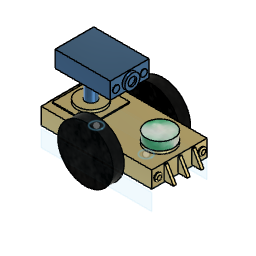
frp_1100309 v2 (Autodesk Fusion 360 design; units mm, degrees)
Autodesk Fusion 360 part; units mm, degrees
sketch "Sketch1" plane through (0, 0, 0) normal (0, 0, 1) x (1, 0, 0)
  line L0 (100, -50) -> (-100, -50)
  line L1 (-100, -50) -> (-100, 50)
  line L2 (-100, 50) -> (100, 50)
  line L3 (100, 50) -> (100, -50)
  line L4 (100, -50) -> (-100, 50) construction
  line L5 (-100, -50) -> (100, 50) construction
  dimension "d1" = 200
  dimension "d2" = 100
  constraint horizontal L0
  constraint perpendicular L0 L1
  constraint parallel L0 L2
  constraint parallel L1 L3
  constraint coincident L4 origin
  constraint coincident L5 origin
  measures "d1" distance of L1.end L2.end
  measures "d2" distance of L0.end L1.end
extrude "Extrude1" add sketch "Sketch1" along normal blind 30 makes body 1
sketch "Sketch2" plane through (0, -50, 0) normal (0, -1, 0) x (1, 0, 0)
  line L0 (-100, 0) -> (100, 0)
  line L1 (100, 0) -> (100, 30)
  line L2 (100, 30) -> (-100, 30)
  line L3 (-100, 30) -> (-100, 0)
sketch "Sketch3" plane through (0, 50, 0) normal (0, 1, 0) x (-1, 0, 0)
  line L0 (-100, 0) -> (100, 0)
  line L1 (100, 0) -> (100, 30)
  line L2 (100, 30) -> (-100, 30)
  line L3 (-100, 30) -> (-100, 0)
  circle A0 centre (0, 15) radius 25
  dimension "d8" = 50
  measures "d8" diameter of A0
sketch "Sketch4" plane through (0, 0, 30) normal (0, 0, 1) x (-1, 0, 0)
  line L0 (-100, -50) -> (100, -50)
  line L1 (100, -50) -> (100, 50)
  line L2 (100, 50) -> (-100, 50)
  line L3 (-100, 50) -> (-100, -50)
  circle A0 centre (-65, 0) radius 25
  dimension "d11" = 50
  measures "d11" diameter of A0
extrude "Extrude4" add sketch "Sketch4" along normal blind 5 contours A0 bodies 1
sketch "Sketch5" plane through (0, 0, 35) normal (0, 0, 1) x (-1, 0, 0)
  circle A0 centre (-65, 0) radius 25
  circle A1 centre (-65, 0) radius 25
  dimension "d14" = 50
  constraint concentric A0 A1
  measures "d14" diameter of A1
extrude "Extrude5" add sketch "Sketch5" along normal blind 15 separate body makes body 2
sketch "Sketch6" plane through (0, 0, 30) normal (0, 0, 1) x (-1, 0, 0)
  circle A0 centre (-65, 0) radius 25
  line L0 (-100, -50) -> (100, -50)
  line L1 (100, -50) -> (100, 50)
  line L2 (100, 50) -> (-100, 50)
  line L3 (-100, 50) -> (-100, -50)
  line L4 (25, 35) -> (95, 35)
  line L5 (95, 35) -> (95, -35)
  line L6 (95, -35) -> (25, -35)
  line L7 (25, -35) -> (25, 35)
  line L8 (25, 35) -> (95, -35) construction
  line L9 (95, 35) -> (25, -35) construction
  point P0 (60, 0)
  dimension "d17" = 70
  dimension "d18" = 70
  constraint horizontal L4
  constraint perpendicular L4 L5
  constraint parallel L4 L6
  constraint parallel L5 L7
  constraint coincident L8 P0
  constraint coincident L9 P0
  measures "d17" distance of L5.end L6.end
  measures "d18" distance of L4.end L5.end
extrude "Extrude6" add sketch "Sketch6" along normal blind 2 contours L4 L5 L6 L7 bodies 1
sketch "Sketch7" plane through (0, 0, 32) normal (0, 0, 1) x (-1, 0, 0)
  line L0 (25, -35) -> (95, -35)
  line L1 (95, -35) -> (95, 35)
  line L2 (95, 35) -> (25, 35)
  line L3 (25, 35) -> (25, -35)
  circle A0 centre (60, 0) radius 25
  dimension "d21" = 50
  measures "d21" diameter of A0
extrude "Extrude7" add sketch "Sketch7" along normal blind 5 contours A0 bodies 1
sketch "Sketch8" plane through (0, 0, 37) normal (0, 0, 1) x (-1, 0, 0)
  circle A0 centre (60, 0) radius 25
  circle A1 centre (60, 0) radius 10
  dimension "d24" = 20
  constraint concentric A0 A1
  measures "d24" diameter of A1
extrude "Extrude8" add sketch "Sketch8" along normal blind 50 separate body contours A1 makes body 3
sketch "Sketch9" plane through (0, 0, 87) normal (0, 0, 1) x (-1, 0, 0)
  circle A0 centre (60, 0) radius 10
  line L0 (-10, -35) -> (90, -35)
  line L1 (90, -35) -> (90, 35)
  line L2 (90, 35) -> (-10, 35)
  line L3 (-10, 35) -> (-10, -35)
  line L4 (-10, -35) -> (90, 35) construction
  line L5 (90, -35) -> (-10, 35) construction
  point P0 (40, 0)
  dimension "d27" = 100
  constraint horizontal L0
  constraint perpendicular L0 L1
  constraint parallel L0 L2
  constraint parallel L1 L3
  constraint coincident L4 P0
  constraint coincident L5 P0
  measures "d27" distance of L1.end L2.end
extrude "Extrude9" add sketch "Sketch9" along normal blind 30 contours A0 | L0 L1 L2 L3 bodies 3
sketch "Sketch10" plane through (10, 0, 0) normal (1, 0, 0) x (0, 1, 0)
  line L0 (-35, 87) -> (35, 87)
  line L1 (35, 87) -> (35, 117)
  line L2 (35, 117) -> (-35, 117)
  line L3 (-35, 117) -> (-35, 87)
  circle A0 centre (0, 101.2139) radius 13.5
  circle A1 centre (-25, 100) radius 6
  circle A2 centre (25, 100) radius 6
  dimension "d30" = 27
  dimension "d31" = 12
  dimension "d32" = 12
  measures "d30" diameter of A0
  measures "d31" diameter of A1
  measures "d32" diameter of A2
extrude "Extrude10" add sketch "Sketch10" along normal blind 2 contours A0 bodies 3
extrude "Extrude11" add sketch "Sketch10" along normal blind 1 contours A1 bodies 3
extrude "Extrude12" add sketch "Sketch10" along normal blind 1 contours A2 bodies 3
sketch "Sketch11" plane through (12, 0, 0) normal (1, 0, 0) x (0, 1, 0)
  circle A0 centre (0, 101.2139) radius 13.5
  circle A1 centre (0, 101.2139) radius 7.5
  dimension "d39" = 15
  constraint concentric A0 A1
  measures "d39" diameter of A1
extrude "Extrude13" add sketch "Sketch11" along normal blind 3 bodies 3
sketch "Sketch12" plane through (100, 0, 0) normal (1, 0, 0) x (0, 1, 0)
  line L0 (-50, 0) -> (50, 0)
  line L1 (50, 0) -> (50, 30)
  line L2 (50, 30) -> (-50, 30)
  line L3 (-50, 30) -> (-50, 0)
  line L4 (-22.5, 2) -> (-27.5, 2)
  line L5 (-27.5, 2) -> (-27.5, 28)
  line L6 (-27.5, 28) -> (-22.5, 28)
  line L7 (-22.5, 28) -> (-22.5, 2)
  line L8 (-22.5, 2) -> (-27.5, 28) construction
  line L9 (-27.5, 2) -> (-22.5, 28) construction
  line L10 (2.5, 2) -> (-2.5, 2)
  line L11 (-2.5, 2) -> (-2.5, 28)
  line L12 (-2.5, 28) -> (2.5, 28)
  line L13 (2.5, 28) -> (2.5, 2)
  line L14 (2.5, 2) -> (-2.5, 28) construction
  line L15 (-2.5, 2) -> (2.5, 28) construction
  line L16 (27.5, 2) -> (22.5, 2)
  line L17 (22.5, 2) -> (22.5, 28)
  line L18 (22.5, 28) -> (27.5, 28)
  line L19 (27.5, 28) -> (27.5, 2)
  line L20 (27.5, 2) -> (22.5, 28) construction
  line L21 (22.5, 2) -> (27.5, 28) construction
  point P0 (-25, 15)
  point P1 (0, 15)
  point P2 (25, 15)
  dimension "d42" = 5
  dimension "d43" = 26
  dimension "d44" = 5
  dimension "d45" = 26
  dimension "d46" = 5
  dimension "d47" = 26
  constraint horizontal L4
  constraint perpendicular L4 L5
  constraint parallel L4 L6
  constraint parallel L5 L7
  constraint coincident L8 P0
  constraint coincident L9 P0
  constraint horizontal L10
  constraint perpendicular L10 L11
  constraint parallel L10 L12
  constraint parallel L11 L13
  constraint coincident L14 P1
  constraint coincident L15 P1
  constraint horizontal L16
  constraint perpendicular L16 L17
  constraint parallel L16 L18
  constraint parallel L17 L19
  constraint coincident L20 P2
  constraint coincident L21 P2
  measures "d42" distance of L5.end L6.end
  measures "d43" distance of L4.end L5.end
  measures "d44" distance of L11.end L12.end
  measures "d45" distance of L10.end L11.end
  measures "d46" distance of L17.end L18.end
  measures "d47" distance of L16.end L17.end
extrude "Extrude14" add sketch "Sketch12" along normal blind 2 contours L4 L5 L6 L7 bodies 1
extrude "Extrude15" add sketch "Sketch12" along normal blind 2 contours L10 L11 L12 L13 bodies 1
extrude "Extrude16" add sketch "Sketch12" along normal blind 2 contours L16 L17 L18 L19 bodies 1
draft "Draft1" angle 30 neutral plane through (100, -27.5, 28) pull (0, 0, 1) 1 faces at (102, -24.1667, 19.3333) on bodies 1
draft "Draft2" angle 30 neutral plane through (100, -2.5, 28) pull (0, 0, 1) 1 faces at (102, -0.8333, 10.6667) on bodies 1
draft "Draft3" angle 30 neutral plane through (100, 22.5, 28) pull (0, 0, 1) 1 faces at (102, 25.8333, 19.3333) on bodies 1
sketch "Sketch13" plane through (100, 0, 0) normal (1, 0, 0) x (0, 1, 0)
  circle A0 centre (-40, 15) radius 6.5
  circle A1 centre (40, 15) radius 6.5
  dimension "d60" = 13
  dimension "d61" = 13
  measures "d60" diameter of A0
  measures "d61" diameter of A1
extrude "Extrude17" add sketch "Sketch13" along normal blind 4 contours A0 bodies 1
extrude "Extrude18" add sketch "Sketch13" along normal blind 4 contours A1 bodies 1
fillet "Fillet1" radius 2.5 tangency weight 1.76356 1 faces at (104, -41.5883, 13.5263) on bodies 1
fillet "Fillet2" radius 2.5 1 faces at (104, 38.4117, 13.5263) on bodies 1
sketch "Sketch14" plane through (-100, 0, 0) normal (-1, 0, 0) x (0, -1, 0)
  line L0 (-50, 0) -> (50, 0)
  line L1 (50, 0) -> (50, 30)
  line L2 (50, 30) -> (-50, 30)
  line L3 (-50, 30) -> (-50, 0)
  line L4 (35, 26.5) -> (-35, 26.5)
  line L5 (-35, 26.5) -> (-35, 3.5)
  line L6 (-35, 3.5) -> (35, 3.5)
  line L7 (35, 3.5) -> (35, 26.5)
  line L8 (35, 26.5) -> (-35, 3.5) construction
  line L9 (-35, 26.5) -> (35, 3.5) construction
  point P0 (0, 15)
  dimension "d70" = 70
  dimension "d71" = 23
  constraint horizontal L4
  constraint perpendicular L4 L5
  constraint parallel L4 L6
  constraint parallel L5 L7
  constraint coincident L8 P0
  constraint coincident L9 P0
  measures "d70" distance of L5.end L6.end
  measures "d71" distance of L4.end L5.end
extrude "Extrude19" add sketch "Sketch14" along normal blind 2 contours L4 L5 L6 L7 bodies 1
sketch "Sketch15" plane through (-102, 0, 0) normal (-1, 0, 0) x (0, -1, 0)
  line L0 (35, 3.5) -> (35, 26.5)
  line L1 (35, 26.5) -> (-35, 26.5)
  line L2 (-35, 26.5) -> (-35, 3.5)
  line L3 (-35, 3.5) -> (35, 3.5)
  line L4 (-18, 6) -> (-22, 6)
  line L5 (-22, 6) -> (-22, 24)
  line L6 (-22, 24) -> (-18, 24)
  line L7 (-18, 24) -> (-18, 6)
  line L8 (-18, 6) -> (-22, 24) construction
  line L9 (-22, 6) -> (-18, 24) construction
  line L10 (2, 24) -> (-2, 24)
  line L11 (-2, 24) -> (-2, 6)
  line L12 (-2, 6) -> (2, 6)
  line L13 (2, 6) -> (2, 24)
  line L14 (2, 24) -> (-2, 6) construction
  line L15 (-2, 24) -> (2, 6) construction
  line L16 (22, 6) -> (18, 6)
  line L17 (18, 6) -> (18, 24)
  line L18 (18, 24) -> (22, 24)
  line L19 (22, 24) -> (22, 6)
  line L20 (22, 6) -> (18, 24) construction
  line L21 (18, 6) -> (22, 24) construction
  point P0 (-20, 15)
  point P1 (0, 15)
  point P2 (20, 15)
  dimension "d74" = 4
  dimension "d75" = 18
  dimension "d76" = 4
  dimension "d77" = 18
  dimension "d78" = 4
  dimension "d79" = 18
  constraint horizontal L4
  constraint perpendicular L4 L5
  constraint parallel L4 L6
  constraint parallel L5 L7
  constraint coincident L8 P0
  constraint coincident L9 P0
  constraint horizontal L10
  constraint perpendicular L10 L11
  constraint parallel L10 L12
  constraint parallel L11 L13
  constraint coincident L14 P1
  constraint coincident L15 P1
  constraint horizontal L16
  constraint perpendicular L16 L17
  constraint parallel L16 L18
  constraint parallel L17 L19
  constraint coincident L20 P2
  constraint coincident L21 P2
  measures "d74" distance of L5.end L6.end
  measures "d75" distance of L4.end L5.end
  measures "d76" distance of L11.end L12.end
  measures "d77" distance of L10.end L11.end
  measures "d78" distance of L17.end L18.end
  measures "d79" distance of L16.end L17.end
extrude "Extrude20" add sketch "Sketch15" along normal blind 2 bodies 1
sketch "Sketch16" plane through (-100, 0, 0) normal (-1, 0, 0) x (0, -1, 0)
  line L0 (35, 3.5) -> (-35, 3.5)
  line L1 (-35, 3.5) -> (-35, 26.5)
  line L2 (-35, 26.5) -> (35, 26.5)
  line L3 (35, 26.5) -> (35, 3.5)
  line L4 (-50, 0) -> (50, 0)
  line L5 (50, 0) -> (50, 30)
  line L6 (50, 30) -> (-50, 30)
  line L7 (-50, 30) -> (-50, 0)
  circle A0 centre (-43, 21) radius 4
  circle A1 centre (43, 21) radius 4
  dimension "d82" = 8
  dimension "d83" = 8
  measures "d82" diameter of A0
  measures "d83" diameter of A1
extrude "Extrude21" add sketch "Sketch16" along normal blind 5 separate body contours A0 makes body 4
extrude "Extrude22" add sketch "Sketch16" along normal blind 5 separate body contours A1 makes body 5
fillet "Fillet3" radius 4 1 faces at (-105, -41.7702, 20.8013) on bodies 5
fillet "Fillet4" radius 4 1 faces at (-105, 44.2298, 20.8013) on bodies 4
ref_plane "WorkPlane1" through (0, -53.7428, -10) normal (0, 0, -1) x (-1, 0, 0)
sketch "Sketch18" plane through (0, 0, 0) normal (0, 0, -1) x (1, 0, 0)
  line L0 (-100, -50) -> (100, -50)
  line L1 (100, -50) -> (100, 50)
  line L2 (100, 50) -> (-100, 50)
  line L3 (-100, 50) -> (-100, -50)
  circle A0 centre (-75, 0) radius 10
  circle A1 centre (65, 0) radius 10
  dimension "d95" = 20
  dimension "d96" = 20
  measures "d95" diameter of A0
  measures "d96" diameter of A1
extrude "Extrude23" add sketch "Sketch18" along normal blind 10 contours A1 bodies 1
extrude "Extrude24" add sketch "Sketch18" along normal blind 10 contours A0 bodies 1
fillet "Fillet5" radius 7.5 1 faces at (-77.5721, -1.414, -10) on bodies 1
fillet "Fillet6" radius 7.5 1 faces at (62.2459, -1.8777, -10) on bodies 1
sketch "Sketch19" plane through (0, -50, 0) normal (0, -1, 0) x (1, 0, 0)
  line L0 (-100, 10) -> (100, 10)
  line L1 (100, 10) -> (100, 40)
  line L2 (100, 40) -> (-100, 40)
  line L3 (-100, 40) -> (-100, 10)
  circle A0 centre (0, 25) radius 50
  dimension "d149" = 100
  measures "d149" diameter of A0
sketch "Sketch20" plane through (0, 50, 0) normal (0, 1, 0) x (-1, 0, 0)
  line L0 (-100, 0) -> (100, 0)
  line L1 (100, 0) -> (100, 30)
  line L2 (100, 30) -> (-100, 30)
  line L3 (-100, 30) -> (-100, 0)
sketch "Sketch21" plane through (0, -50, 0) normal (0, -1, 0) x (1, 0, 0)
  circle A0 centre (0, 15) radius 50
  dimension "d152" = 100
  measures "d152" diameter of A0
extrude "Extrude26" add sketch "Sketch21" along normal blind 20 separate body makes body 6
sketch "Sketch22" plane through (0, 50, 0) normal (0, 1, 0) x (-1, 0, 0)
  circle A0 centre (0, 15) radius 50
  dimension "d155" = 100
  measures "d155" diameter of A0
extrude "Extrude27" add sketch "Sketch22" along normal blind 20 separate body makes body 7
ref_plane "WorkPlane2" through (0, 50.0691, -35) normal (0, 0, -1) x (1, 0, 0)
move_body "Move2" bodies 7 6 1 3 2 4 5 to x (1, 0, 0) y (0, 1, 0) z (0, 0, 1) at (0, 0, 35)
sketch "Sketch25" plane through (0, 0, 35) normal (0, 0, -1) x (1, 0, 0)
  circle A0 centre (-75, 0) radius 10
  circle A1 centre (65, 0) radius 10
  line L0 (-100, -50) -> (100, -50)
  line L1 (100, -50) -> (100, 50)
  line L2 (100, 50) -> (-100, 50)
  line L3 (-100, 50) -> (-100, -50)
sketch "Sketch26" plane through (0, 0, 35) normal (0, 0, -1) x (1, 0, 0)
  circle A0 centre (40, 0) radius 10
  circle A1 centre (-50, 0) radius 10
  dimension "d161" = 20
  dimension "d162" = 20
  measures "d161" diameter of A0
  measures "d162" diameter of A1
extrude "Extrude28" add sketch "Sketch26" along normal blind 35 contours A0 bodies 1
extrude "Extrude29" add sketch "Sketch26" along normal blind 35 contours A1 bodies 1
fillet "Fillet7" radius 10 1 faces at (37.5193, 1.7704, 0) on bodies 1
fillet "Fillet8" radius 10 1 faces at (-47.4279, 0.5511, 0) on bodies 1
copy_body "Body->Comp8" bodies 1 removing the originals makes body 8 in component "base_link"
copy_body "Body->Comp9" bodies 2 removing the originals makes body 9 in component "lidar"
copy_body "Body->Comp10" bodies 3 removing the originals makes body 10 in component "camera"
copy_body "Body->Comp11" bodies 4 removing the originals makes body 11 in component "left_light"
copy_body "Body->Comp12" bodies 5 removing the originals makes body 12 in component "right_light"
copy_body "Body->Comp13" bodies 6 removing the originals makes body 13 in component "right_wheel"
copy_body "Body->Comp14" bodies 7 removing the originals makes body 14 in component "left_wheel"
component "base_link" placed x (1, 0, 0) y (0, 1, 0) z (0, 0, 1) at (0, 0, 0)
component "lidar" placed x (1, 0, 0) y (0, 1, 0) z (0, 0, 1) at (0, 0, 0)
component "camera" placed x (1, 0, 0) y (0, 1, 0) z (0, 0, 1) at (0, 0, 0)
component "left_light" placed x (1, 0, 0) y (0, 1, 0) z (0, 0, 1) at (0, 0, 0)
component "right_light" placed x (1, 0, 0) y (0, 1, 0) z (0, 0, 1) at (0, 0, 0)
component "right_wheel" placed x (1, 0, 0) y (0, 1, 0) z (0, 0, 1) at (0, 0, 0)
component "left_wheel" placed x (1, 0, 0) y (0, 1, 0) z (0, 0, 1) at (0, 0, 0)
named bodies: "base_link", "lidar", "camera", "left_light", "right_light", "right_wheel", "left_wheel"
